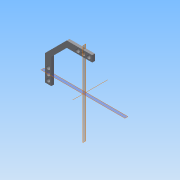
# Autodesk Inventor part: renfort
Saved by Autodesk Inventor 2015 (Build 190159000, 159)
## iProperties
Created: 2015-06-18
Part Number: renfort
Material: Générique
Document SubType Name: Modeling
Designer: Gregwar
Density: 1 g/cm^3
Appearance: Par défaut
Author: Gregwar
Autodesk Inventor part; units mm, degrees
ref_plane "YZ Plane" through (0, 0, 0) normal (1, 0, 0) x (0, 1, 0)
ref_plane "XZ Plane" through (0, 0, 0) normal (0, 1, 0) x (-1, 0, 0)
ref_plane "XY Plane" through (0, 0, 0) normal (0, 0, 1) x (1, 0, 0)
sketch "Esquisse1" plane through (0, 0, 0) normal (0, 1, 0) x (-1, 0, 0)
  line L0 (35, 35) -> (35, 14)
  line L1 (35, 14) -> (42, 10)
  line L2 (42, 10) -> (42, 0)
  line L3 (35, 35) -> (0, 0)
  line L4 (42, 0) -> (0, 0) construction
  line L5 (35, -35) -> (35, -14)
  line L6 (35, -14) -> (42, -10)
  line L7 (42, -10) -> (42, 0)
  line L8 (35, -35) -> (0, 0)
  line L9 (38.5, -12) -> (38.5, 12) construction
  circle A0 centre (38.5, 0) radius 2.15
  circle A1 centre (38.5, 6) radius 2.15
  circle A2 centre (38.5, -6) radius 2.15
  dimension "d0" = 90
  dimension "d1" = 70
  dimension "d4" = 6
  dimension "d11" = 6
  dimension "d16" = 4.3
  dimension "d17" = 20
  dimension "d18" = 4
  dimension "d19" = 7
  constraints: 20 end point, 3 centre point, 3 midpoint, 3 symmetric about line, 3 vertical, 1 horizontal, 1 parallel, 4 other
  measures "d0" angle of L3 L8
  measures "d1" distance of L0.start L5.start
  measures "d4" distance of A0.centre A1.centre
  measures "d11" distance of A0.centre A2.centre
  measures "d16" diameter of A0
  measures "d17" distance of L1.end L6.end
  measures "d18" vertical distance of L1.end L0.end
  measures "d19" distance between parallel lines of L5 L7
extrude "Extrusion1" add sketch "Esquisse1" along normal blind 3
pattern_circular "Réseau circulaire1" count 4 over 360 about axis through (0, 0, 0) along (0, 1, 0) of "Extrusion1"
ref_plane "Plan de construction2" through (0, 0, -14) normal (1, 0, 0) x (0, 0, -1)
ref_plane "Plan de construction3" through (-14, 0, 0) normal (0, 0, -1) x (-1, 0, 0)
chamfer "Chanfrein1" distance 10 angle 45 4 edges at (-35, 1.5, -35) (-35, 1.5, 35) (35, 1.5, -35) (35, 1.5, 35)
sketch "Esquisse3" plane through (0, 0, 0) normal (0, -1, 0) x (1, 0, 0)
  circle A0 centre (0, 38.5) radius 2.15 construction
  circle A1 centre (6, 38.5) radius 2.15 construction
  circle A2 centre (-6, 38.5) radius 2.15 construction
  circle A3 centre (38.5, 6) radius 2.15 construction
  circle A4 centre (38.5, -6) radius 2.15 construction
  circle A5 centre (38.5, 0) radius 2.15 construction
  circle A6 centre (6, -38.5) radius 2.15 construction
  circle A7 centre (-6, -38.5) radius 2.15 construction
  circle A8 centre (0, -38.5) radius 2.15 construction
  circle A9 centre (-38.5, -6) radius 2.15 construction
  circle A10 centre (-38.5, 6) radius 2.15 construction
  circle A11 centre (-38.5, 0) radius 2.15 construction
  line L0 (-35, 25) -> (-35, 14) construction
  line L1 (-35, 14) -> (-42, 10) construction
  line L2 (-42, 10) -> (-42, -10) construction
  line L3 (-42, -10) -> (-35, -14) construction
  line L4 (-35, -14) -> (-35, -25) construction
  line L5 (-25, -35) -> (-14, -35) construction
  line L6 (-14, -35) -> (-10, -42) construction
  line L7 (-10, -42) -> (10, -42) construction
  line L8 (10, -42) -> (14, -35) construction
  line L9 (14, -35) -> (25, -35) construction
  line L10 (35, -25) -> (35, -14) construction
  line L11 (35, -14) -> (42, -10) construction
  line L12 (42, -10) -> (42, 10) construction
  line L13 (42, 10) -> (35, 14) construction
  line L14 (35, 14) -> (35, 25) construction
  line L15 (25, 35) -> (14, 35) construction
  line L16 (14, 35) -> (10, 42) construction
  line L17 (10, 42) -> (-10, 42) construction
  line L18 (-10, 42) -> (-14, 35) construction
  line L19 (-14, 35) -> (-25, 35) construction
  line L20 (-51.72, -12.8291) -> (-12.8291, -51.72)
  line L21 (-12.8291, -51.72) -> (-10, -42)
  line L22 (-42, -10) -> (-51.72, -12.8291)
  line L23 (-35, -14) -> (-42, -10)
  line L24 (-42, -10) -> (-35, -14) projected
  line L25 (-10, -42) -> (-14, -35)
  line L26 (-14, -35) -> (-10, -42) projected
  line L27 (25, 35) -> (35, 25) projected
  line L28 (-35, 25) -> (-25, 35) projected
  line L29 (-25, -35) -> (-35, -25) projected
  line L30 (35, -25) -> (25, -35) projected
  line L31 (-14, -35) -> (-35, -14)
  point P0 (0, 0)
  dimension "d32" = 135
  dimension "d33" = 55
  constraints: 12 end point, 1 collinear, 1 equal length, 1 point on line
  measures "d32" angle of L5 L20
  measures "d33" distance of L20.start L20.end
extrude "Extrusion3" add sketch "Esquisse3" against normal blind 3
sketch "Esquisse4" plane through (-51.72, 0, -12.8291) normal (-0.7071, 0, -0.7071) x (-0.7071, 0, 0.7071)
  line L0 (0, 0) -> (-55, 0) construction
  line L1 (0, 0) -> (0, 3) construction
  line L2 (-55, 3) -> (0, 3) construction
  line L3 (-55, 0) -> (-55, 3) construction
  line L4 (0, 0) -> (-55, 0)
  line L5 (-55, 0) -> (-55, 24)
  line L6 (-55, 24) -> (0, 24)
  line L7 (0, 24) -> (0, 0)
  point P0 (-27.5, 0)
  dimension "d36" = 24
  constraints: 8 end point, 2 parallel, 1 horizontal, 1 perpendicular
  measures "d36" distance of L4.end L5.end
extrude "Extrusion4" add sketch "Esquisse4" along normal blind 3
sketch "Esquisse5" plane through (-53.8413, 0, -14.9504) normal (-0.7071, 0, -0.7071) x (-0.7071, 0, 0.7071)
  line L0 (-55, 0) -> (0, 0) construction
  line L1 (0, 0) -> (0, 24) construction
  line L2 (0, 24) -> (-55, 24) construction
  line L3 (-55, 24) -> (-55, 0) construction
  line L4 (0, 0) -> (0, 24) construction
  line L5 (0, 9.2801) -> (-55, 9.2801) construction
  circle A0 centre (-15.1412, 9.2801) radius 7.3571
  line L6 (-27.5, 0) -> (-27.5, 24) construction
  circle A1 centre (-39.8588, 9.2801) radius 7.3571
  constraints: 4 end point, 3 point on line, 2 centre point, 1 midpoint, 1 perpendicular, 1 symmetric about line, 1 other
extrude "Extrusion5" cut sketch "Esquisse5" against normal blind 1
pattern_circular "Réseau circulaire2" count 4 over 360 about axis through (0, 0, 0) along (0, -1, 0) of "Extrusion3", "Extrusion4"
fillet "Congé1" radius 3 2 edges at (-34.3959, 0, 34.3959) (34.3959, 0, -34.3959)
sketch "Esquisse13" plane through (0, 3, 0) normal (0, 1, 0) x (1, 0, 0)
  line L0 (-10, -42) -> (10, -42) construction
  line L1 (10, -42) -> (12.8291, -51.72) construction
  line L2 (12.8291, -51.72) -> (51.72, -12.8291) construction
  line L3 (51.72, -12.8291) -> (42, -10) construction
  line L4 (42, -10) -> (42, 10) construction
  line L5 (42, 10) -> (51.72, 12.8291) construction
  line L6 (51.72, 12.8291) -> (12.8291, 51.72) construction
  line L7 (12.8291, 51.72) -> (10, 42) construction
  line L8 (10, 42) -> (-10, 42) construction
  line L9 (-10, 42) -> (-12.8291, 51.72) construction
  line L10 (-12.8291, 51.72) -> (-51.72, 12.8291) construction
  line L11 (-51.72, 12.8291) -> (-42, 10) construction
  line L12 (-42, 10) -> (-42, -10) construction
  line L13 (-42, -10) -> (-51.72, -12.8291) construction
  line L14 (-51.72, -12.8291) -> (-12.8291, -51.72) construction
  line L15 (-12.8291, -51.72) -> (-10, -42) construction
  circle A0 centre (0, -38.5) radius 2.15 construction
  circle A1 centre (6, -38.5) radius 2.15 construction
  circle A2 centre (-6, -38.5) radius 2.15 construction
  circle A3 centre (38.5, -6) radius 2.15 construction
  circle A4 centre (38.5, 6) radius 2.15 construction
  circle A5 centre (38.5, 0) radius 2.15 construction
  circle A6 centre (6, 38.5) radius 2.15 construction
  circle A7 centre (-6, 38.5) radius 2.15 construction
  circle A8 centre (0, 38.5) radius 2.15 construction
  circle A9 centre (-38.5, 6) radius 2.15 construction
  circle A10 centre (-38.5, -6) radius 2.15 construction
  circle A11 centre (-38.5, 0) radius 2.15 construction
  line L16 (10, -42) -> (-18, -42)
  line L17 (-18, -42) -> (-42, -18)
  line L18 (-42, -18) -> (-42, 10)
  line L19 (-42, -10) -> (-42, 10) projected
  line L20 (-42, 10) -> (-35, 10)
  line L21 (-35, 10) -> (-35, -17.9289)
  line L22 (-35, -17.9289) -> (-17.9289, -35)
  line L23 (-17.9289, -35) -> (10, -35)
  line L24 (10, -35) -> (10, -42)
  line L25 (-10, -42) -> (10, -42) projected
  dimension "d97" = 7
  dimension "d98" = 5
  dimension "d99" = 28
  constraints: 16 end point, 5 perpendicular, 2 collinear, 2 parallel
  measures "d97" distance of L11.end L20.end
  measures "d98" distance between parallel lines of L17 L22
  measures "d99" distance of L17.end L11.end
extrude "Extrusion11" cut sketch "Esquisse13" against normal blind 10 keep common part
